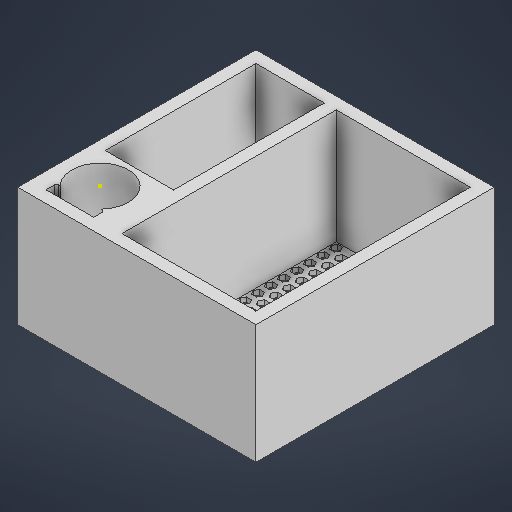
# Autodesk Inventor part: mount
Saved by Autodesk Inventor 2026.1 (Build 301233020, 233B)
## iProperties
Created: 2025-12-18
Part Number: mount
Material: Generic
Document SubType Name: Modeling
Designer: Fish
Density: 1 g/cm^3
Appearance: Default
Author: Fish
Autodesk Inventor part; units mm, degrees
(part 1 of 4)
ref_plane "YZ Plane" through (0, 0, 0) normal (1, 0, 0) x (0, 1, 0)
ref_plane "XZ Plane" through (0, 0, 0) normal (0, 1, 0) x (-1, 0, 0)
ref_plane "XY Plane" through (0, 0, 0) normal (0, 0, 1) x (1, 0, 0)
sketch "Sketch1" plane through (0, 0, 0) normal (0, 1, 0) x (-1, 0, 0)
  circle A0 centre (0, 0) radius 11.5
  circle A1 centre (0, 0) radius 11.85
  line L0 (10, 12.5) -> (-10, 12.5)
  line L1 (-10, 12.5) -> (-10, 8.2614)
  line L2 (-10, 8.2614) -> (10, 8.2614)
  line L3 (10, 8.2614) -> (10, 12.5)
  line L4 (10, 12.5) -> (-10, 8.2614) construction
  line L5 (-10, 12.5) -> (10, 8.2614) construction
  line L6 (0, 10.3807) -> (0, -11.5) construction
  line L7 (10, 12.5) -> (-10, 12.5)
  line L8 (-10, 12.5) -> (-10, 12.7)
  line L9 (-10, 12.7) -> (10, 12.7)
  line L10 (10, 12.7) -> (10, 12.5)
  line L11 (-16.85, 17.7) -> (16.85, 17.7)
  line L12 (16.85, 17.7) -> (16.85, -14)
  line L13 (16.85, -14) -> (-16.85, -14)
  line L14 (-16.85, -14) -> (-16.85, 17.7)
  point P0 (8, 8.2614)
  point P1 (-8, 8.2614)
  point P2 (0, -14)
  point P3 (8.4954, 8.2614)
  point P4 (-8.4954, 8.2614)
  dimension "d0" = 23
  dimension "d1" = 0.35
  dimension "d2" = 24
  dimension "d3" = 16
  dimension "d4" = 20
  dimension "d5" = 0.2
  dimension "d6" = 5
  dimension "d7" = 2.5
  dimension "d8" = 5
  dimension "d9" = 16.85
  dimension "d10" = 16.85
  constraints: 30 end point, 6 parallel, 3 horizontal, 3 midpoint, 3 perpendicular, 3 point on circle, 3 point on line, 2 centre point, 2 coincident, 1 vertical
  measures "d0" diameter of A0
  measures "d1" radial gap between concentric circles of A1 A0
  measures "d2" distance from line of L0 L6.end
  measures "d3" distance of point (-8, 8.261) A0.end
  measures "d4" distance of L0.start L0.end
  measures "d5" distance between parallel lines of L9 L0
  measures "d6" distance between parallel lines of L11 L9
  measures "d7" distance of point (0, -14) L6.end
  measures "d8" distance edge to line of A1 L14
  measures "d9" distance between parallel lines of L14 L6
  measures "d10" distance between parallel lines of L12 L6
extrude "Extrusion1" add sketch "Sketch1" along normal blind 50
fillet "Fillet1" radius 0.25 2 edges at (8.4954, 25, 8.2614) (-8.4954, 25, 8.2614)
chamfer "Chamfer1" distance 0.75 angle 45 2 edges at (-10, 25, 8.2614) (10, 25, 8.2614)
sketch "Sketch2" plane through (16.85, 0, -14) normal (0, 0, -1) x (-1, 0, 0)
  line L0 (5, 50) -> (28.7, 50) projected
  line L1 (5, 50) -> (28.7, 50)
  line L2 (28.7, 50) -> (28.7, 0)
  line L3 (28.7, 0) -> (5, 0)
  line L4 (5, 0) -> (5, 50)
  line L5 (0, 0) -> (33.7, 0) projected
  circle A0 centre (8.8, 2.3324) radius 3.5
  circle A1 centre (8.8, 2.3324) radius 3.8
  line L6 (5.8, 0) -> (11.8, 0) construction
  line L7 (5.3, 0) -> (5.3, 50)
  point P0 (16.85, 0)
  point P1 (25.7306, 50)
  point P2 (7.9694, 50)
  point P3 (2.5, 2.3324)
  point P4 (6.1904, 0)
  point P5 (11.8, 0)
  point P6 (5, 2.3324)
  point P7 (2.5, 0.8525)
  point P8 (11.4096, 0)
  dimension "d17" = 7
  dimension "d18" = 0.3
  dimension "d20" = 6
  dimension "d25" = 0.3
  constraints: 12 end point, 4 point on line, 2 centre point, 2 horizontal, 2 parallel, 2 perpendicular, 2 point on circle, 1 coincident, 1 tangent
  measures "d17" diameter of A0
  measures "d18" radial gap between concentric circles of A1 A0
  measures "d20" distance of L6.end L6.start
  measures "d25" distance between parallel lines of L4 L7
extrude "Extrusion2" cut sketch "Sketch2" against normal up to surface contours A1 L7 | A1 L3 A0 L7 | L7 A0 L3 A1 | A0 L3 | L3 A0 A1 | L3 A0
fillet "Fillet2" radius 0.25 2 edges at (5.05, 0, -12.36) (11.05, 0, -9.1401)
sketch "Sketch4" plane through (16.85, 50, -14) normal (0, 0, -1) x (-1, 0, 0)
  arc A0 (5.3264, -50) -> (5.5408, -49.6215) centre (5.3264, -49.75) ccw projected
  arc A1 (12.0592, -49.6215) -> (5.5408, -49.6215) centre (8.8, -47.6676) ccw projected
  arc A2 (12.0592, -49.6215) -> (12.2736, -50) centre (12.2736, -49.75) ccw projected
  line L0 (12.2736, -50) -> (33.7, -50) projected
  line L1 (33.7, -50) -> (33.7, 0) projected
  line L2 (0, 0) -> (33.7, 0) projected
  line L3 (0, -50) -> (0, 0) projected
  line L4 (0, -50) -> (5.3264, -50) projected
  line L5 (5.5764, -49.0955) -> (12.0236, -49.0955)
  line L6 (12.0236, -49.0955) -> (12.0236, -49.986)
  line L7 (12.0236, -49.986) -> (5.5764, -49.986)
  line L8 (5.5764, -49.986) -> (5.5764, -49.0955)
  arc A3 (12.0592, -49.6215) -> (12.2736, -50) centre (12.2736, -49.75) ccw projected
  point P0 (16.85, -50)
  dimension "d26" = 6.4473
  constraints: 8 end point, 2 parallel, 2 tangent, 1 horizontal, 1 perpendicular
  measures "d26" distance of L5.start L5.end
sketch "Sketch5" plane through (0, 50, 0) normal (0, 1, 0) x (1, 0, 0)
  point P0 (0, 0)
sketch "Sketch6" plane through (0, 50, 0) normal (0, 1, 0) x (1, 0, 0)
  line L0 (-16.85, -17.7) -> (16.85, -17.7) projected
  line L1 (-16.85, -17.7) -> (83.15, -17.7)
  line L2 (83.15, -17.7) -> (83.15, 82.3)
  line L3 (83.15, 82.3) -> (-16.85, 82.3)
  line L4 (-16.85, 82.3) -> (-16.85, -17.7)
  line L5 (16.85, -17.7) -> (16.85, 14) projected
  line L6 (16.85, -17.7) -> (21.85, -17.7)
  line L7 (21.85, -17.7) -> (21.85, 82.3)
  line L8 (21.85, 82.3) -> (16.85, 82.3)
  line L9 (16.85, 82.3) -> (16.85, -17.7)
  line L10 (21.85, -17.7) -> (83.15, -17.7)
  line L11 (83.15, -17.7) -> (83.15, -12.7)
  line L12 (83.15, -12.7) -> (21.85, -12.7)
  line L13 (21.85, -12.7) -> (21.85, -17.7)
  line L14 (21.85, 82.3) -> (83.15, 82.3)
  line L15 (83.15, 82.3) -> (83.15, 77.3)
  line L16 (83.15, 77.3) -> (21.85, 77.3)
  line L17 (21.85, 77.3) -> (21.85, 82.3)
  line L18 (83.15, -12.7) -> (78.15, -12.7)
  line L19 (78.15, -12.7) -> (78.15, 77.3)
  line L20 (78.15, 77.3) -> (83.15, 77.3)
  line L21 (83.15, 77.3) -> (83.15, -12.7)
  line L22 (16.85, 14) -> (-16.85, 14) projected
  line L23 (-16.85, 14) -> (-11.85, 14)
  line L24 (-11.85, 14) -> (-11.85, 82.3)
  line L25 (-11.85, 82.3) -> (-16.85, 82.3)
  line L26 (-16.85, 82.3) -> (-16.85, 14)
  line L27 (-11.85, 82.3) -> (21.85, 82.3)
  line L28 (21.85, 82.3) -> (21.85, 77.3)
  line L29 (21.85, 77.3) -> (-11.85, 77.3)
  line L30 (-11.85, 77.3) -> (-11.85, 82.3)
  point P0 (0, 0)
  point P1 (-11.85, 77.3)
  point P2 (16.85, 77.3)
  point P3 (16.85, -17.7)
  dimension "d29" = 5
  dimension "d30" = 5
  dimension "d31" = 100
  dimension "d32" = 100
  dimension "d33" = 5
  dimension "d34" = 5
  dimension "d35" = 5
  constraints: 56 end point, 14 parallel, 7 horizontal, 7 perpendicular, 5 point on line
  measures "d29" distance between parallel lines of L7 L9
  measures "d30" distance between parallel lines of L1 L12
  measures "d31" distance of L3.end L0.start
  measures "d32" distance of L2.end L3.end
  measures "d33" distance between parallel lines of L3 L16
  measures "d34" distance between parallel lines of L21 L19
  measures "d35" distance between parallel lines of L4 L24
extrude "Extrusion3" add sketch "Sketch6" against normal up to surface (50 mm away) contours L5 L9 L29 L7 L1 | L4 L3 L24 L22 | L7 L12 L2 L1 | L29 L24 L3 L9 | L9 L3 L7 L29 | L12 L19 L16 L2 | L7 L3 L2 L16
sketch "Sketch7" plane through (0, 0, 0) normal (0, -1, 0) x (1, 0, 0)
  line L0 (21.85, -77.3) -> (21.85, 12.7) projected
  line L1 (21.85, 12.7) -> (78.15, 12.7) projected
  line L2 (78.15, 12.7) -> (78.15, -77.3) projected
  line L3 (78.15, -77.3) -> (21.85, -77.3) projected
  line L4 (20.35, 16.9321) -> (21.35, 15.2)
  line L5 (21.35, 15.2) -> (20.35, 13.4679)
  line L6 (20.35, 13.4679) -> (18.35, 13.4679)
  line L7 (18.35, 13.4679) -> (17.35, 15.2)
  line L8 (17.35, 15.2) -> (18.35, 16.9321)
  line L9 (18.35, 16.9321) -> (20.35, 16.9321)
  line L10 (-16.85, 17.7) -> (83.15, 17.7) projected
  line L11 (25.0821, 19.6641) -> (26.0821, 17.9321)
  line L12 (26.0821, 17.9321) -> (25.0821, 16.2)
  line L13 (25.0821, 16.2) -> (23.0821, 16.2)
  line L14 (23.0821, 16.2) -> (22.0821, 17.9321)
  line L15 (22.0821, 17.9321) -> (23.0821, 19.6641)
  line L16 (23.0821, 19.6641) -> (25.0821, 19.6641)
  line L17 (29.8141, 16.9321) -> (30.8141, 15.2)
  line L18 (30.8141, 15.2) -> (29.8141, 13.4679)
  line L19 (29.8141, 13.4679) -> (27.8141, 13.4679)
  line L20 (27.8141, 13.4679) -> (26.8141, 15.2)
  line L21 (26.8141, 15.2) -> (27.8141, 16.9321)
  line L22 (27.8141, 16.9321) -> (29.8141, 16.9321)
  line L23 (20.35, 16.9321) -> (22.0821, 17.9321) construction
  line L24 (25.0821, 16.2) -> (26.8141, 15.2) construction
  line L25 (25.0821, 14.2) -> (26.0821, 12.4679)
  line L26 (26.0821, 12.4679) -> (25.0821, 10.7359)
  line L27 (25.0821, 10.7359) -> (23.0821, 10.7359)
  line L28 (23.0821, 10.7359) -> (22.0821, 12.4679)
  line L29 (22.0821, 12.4679) -> (23.0821, 14.2)
  line L30 (23.0821, 14.2) -> (25.0821, 14.2)
  line L31 (20.35, 11.4679) -> (21.35, 9.7359)
  line L32 (21.35, 9.7359) -> (20.35, 8.0038)
  line L33 (20.35, 8.0038) -> (18.35, 8.0038)
  line L34 (18.35, 8.0038) -> (17.35, 9.7359)
  line L35 (17.35, 9.7359) -> (18.35, 11.4679)
  line L36 (18.35, 11.4679) -> (20.35, 11.4679)
  line L37 (18.35, 13.4679) -> (18.35, 11.4679) construction
  line L38 (27.8141, 13.4679) -> (26.8141, 15.2)
  line L39 (30.8141, 15.2) -> (29.8141, 13.4679)
  line L40 (27.8141, 16.9321) -> (29.8141, 16.9321)
  line L41 (29.8141, 16.9321) -> (30.8141, 15.2)
  line L42 (29.8141, 13.4679) -> (27.8141, 13.4679)
  line L43 (26.8141, 15.2) -> (27.8141, 16.9321)
  line L44 (32.5462, 16.2) -> (31.5462, 17.9321)
  line L45 (34.5462, 16.2) -> (32.5462, 16.2)
  line L46 (35.5462, 17.9321) -> (34.5462, 16.2)
  line L47 (31.5462, 17.9321) -> (32.5462, 19.6641)
  line L48 (32.5462, 19.6641) -> (34.5462, 19.6641)
  line L49 (34.5462, 19.6641) -> (35.5462, 17.9321)
  line L50 (37.2782, 13.4679) -> (36.2782, 15.2)
  line L51 (40.2782, 15.2) -> (39.2782, 13.4679)
  line L52 (37.2782, 16.9321) -> (39.2782, 16.9321)
  line L53 (39.2782, 16.9321) -> (40.2782, 15.2)
  line L54 (39.2782, 13.4679) -> (37.2782, 13.4679)
  line L55 (36.2782, 15.2) -> (37.2782, 16.9321)
  line L56 (42.0103, 16.2) -> (41.0103, 17.9321)
  line L57 (44.0103, 16.2) -> (42.0103, 16.2)
  line L58 (45.0103, 17.9321) -> (44.0103, 16.2)
  line L59 (41.0103, 17.9321) -> (42.0103, 19.6641)
  line L60 (42.0103, 19.6641) -> (44.0103, 19.6641)
  line L61 (44.0103, 19.6641) -> (45.0103, 17.9321)
  line L62 (46.7423, 13.4679) -> (45.7423, 15.2)
  line L63 (49.7423, 15.2) -> (48.7423, 13.4679)
  line L64 (46.7423, 16.9321) -> (48.7423, 16.9321)
  line L65 (48.7423, 16.9321) -> (49.7423, 15.2)
  line L66 (48.7423, 13.4679) -> (46.7423, 13.4679)
  line L67 (45.7423, 15.2) -> (46.7423, 16.9321)
  line L68 (51.4744, 16.2) -> (50.4744, 17.9321)
  line L69 (53.4744, 16.2) -> (51.4744, 16.2)
  line L70 (54.4744, 17.9321) -> (53.4744, 16.2)
  line L71 (50.4744, 17.9321) -> (51.4744, 19.6641)
  line L72 (51.4744, 19.6641) -> (53.4744, 19.6641)
  line L73 (53.4744, 19.6641) -> (54.4744, 17.9321)
  line L74 (56.2064, 13.4679) -> (55.2064, 15.2)
  line L75 (59.2064, 15.2) -> (58.2064, 13.4679)
  line L76 (56.2064, 16.9321) -> (58.2064, 16.9321)
  line L77 (58.2064, 16.9321) -> (59.2064, 15.2)
  line L78 (58.2064, 13.4679) -> (56.2064, 13.4679)
  line L79 (55.2064, 15.2) -> (56.2064, 16.9321)
  line L80 (60.9385, 16.2) -> (59.9385, 17.9321)
  line L81 (62.9385, 16.2) -> (60.9385, 16.2)
  line L82 (63.9385, 17.9321) -> (62.9385, 16.2)
  line L83 (59.9385, 17.9321) -> (60.9385, 19.6641)
  line L84 (60.9385, 19.6641) -> (62.9385, 19.6641)
  line L85 (62.9385, 19.6641) -> (63.9385, 17.9321)
  line L86 (65.6705, 13.4679) -> (64.6705, 15.2)
  line L87 (68.6705, 15.2) -> (67.6705, 13.4679)
  line L88 (65.6705, 16.9321) -> (67.6705, 16.9321)
  line L89 (67.6705, 16.9321) -> (68.6705, 15.2)
  line L90 (67.6705, 13.4679) -> (65.6705, 13.4679)
  line L91 (64.6705, 15.2) -> (65.6705, 16.9321)
  line L92 (70.4026, 16.2) -> (69.4026, 17.9321)
  line L93 (72.4026, 16.2) -> (70.4026, 16.2)
  line L94 (73.4026, 17.9321) -> (72.4026, 16.2)
  line L95 (69.4026, 17.9321) -> (70.4026, 19.6641)
  line L96 (70.4026, 19.6641) -> (72.4026, 19.6641)
  line L97 (72.4026, 19.6641) -> (73.4026, 17.9321)
  line L98 (75.1346, 13.4679) -> (74.1346, 15.2)
  line L99 (78.1346, 15.2) -> (77.1346, 13.4679)
  line L100 (75.1346, 16.9321) -> (77.1346, 16.9321)
  line L101 (77.1346, 16.9321) -> (78.1346, 15.2)
  line L102 (77.1346, 13.4679) -> (75.1346, 13.4679)
  line L103 (74.1346, 15.2) -> (75.1346, 16.9321)
  line L104 (79.8667, 16.2) -> (78.8667, 17.9321)
  line L105 (81.8667, 16.2) -> (79.8667, 16.2)
  line L106 (82.8667, 17.9321) -> (81.8667, 16.2)
  line L107 (78.8667, 17.9321) -> (79.8667, 19.6641)
  line L108 (79.8667, 19.6641) -> (81.8667, 19.6641)
  line L109 (81.8667, 19.6641) -> (82.8667, 17.9321)
  line L110 (18.35, 8.0038) -> (17.35, 9.7359)
  line L111 (21.35, 9.7359) -> (20.35, 8.0038)
  line L112 (18.35, 11.4679) -> (20.35, 11.4679)
  line L113 (20.35, 11.4679) -> (21.35, 9.7359)
  line L114 (20.35, 8.0038) -> (18.35, 8.0038)
  line L115 (17.35, 9.7359) -> (18.35, 11.4679)
  line L116 (23.0821, 10.7359) -> (22.0821, 12.4679)
  line L117 (25.0821, 10.7359) -> (23.0821, 10.7359)
  line L118 (26.0821, 12.4679) -> (25.0821, 10.7359)
  line L119 (22.0821, 12.4679) -> (23.0821, 14.2)
  line L120 (23.0821, 14.2) -> (25.0821, 14.2)
  line L121 (25.0821, 14.2) -> (26.0821, 12.4679)
  line L122 (27.8141, 8.0038) -> (26.8141, 9.7359)
  line L123 (30.8141, 9.7359) -> (29.8141, 8.0038)
  line L124 (27.8141, 11.4679) -> (29.8141, 11.4679)
  line L125 (29.8141, 11.4679) -> (30.8141, 9.7359)
  line L126 (29.8141, 8.0038) -> (27.8141, 8.0038)
  line L127 (26.8141, 9.7359) -> (27.8141, 11.4679)
  line L128 (32.5462, 10.7359) -> (31.5462, 12.4679)
  line L129 (34.5462, 10.7359) -> (32.5462, 10.7359)
  line L130 (35.5462, 12.4679) -> (34.5462, 10.7359)
  line L131 (31.5462, 12.4679) -> (32.5462, 14.2)
  line L132 (32.5462, 14.2) -> (34.5462, 14.2)
  line L133 (34.5462, 14.2) -> (35.5462, 12.4679)
  line L134 (37.2782, 8.0038) -> (36.2782, 9.7359)
  line L135 (40.2782, 9.7359) -> (39.2782, 8.0038)
  line L136 (37.2782, 11.4679) -> (39.2782, 11.4679)
  line L137 (39.2782, 11.4679) -> (40.2782, 9.7359)
  line L138 (39.2782, 8.0038) -> (37.2782, 8.0038)
  line L139 (36.2782, 9.7359) -> (37.2782, 11.4679)
  line L140 (42.0103, 10.7359) -> (41.0103, 12.4679)
  line L141 (44.0103, 10.7359) -> (42.0103, 10.7359)
  line L142 (45.0103, 12.4679) -> (44.0103, 10.7359)
  line L143 (41.0103, 12.4679) -> (42.0103, 14.2)
  line L144 (42.0103, 14.2) -> (44.0103, 14.2)
  line L145 (44.0103, 14.2) -> (45.0103, 12.4679)
  line L146 (46.7423, 8.0038) -> (45.7423, 9.7359)
  line L147 (49.7423, 9.7359) -> (48.7423, 8.0038)
  line L148 (46.7423, 11.4679) -> (48.7423, 11.4679)
  line L149 (48.7423, 11.4679) -> (49.7423, 9.7359)
  line L150 (48.7423, 8.0038) -> (46.7423, 8.0038)
  line L151 (45.7423, 9.7359) -> (46.7423, 11.4679)
  line L152 (51.4744, 10.7359) -> (50.4744, 12.4679)
  line L153 (53.4744, 10.7359) -> (51.4744, 10.7359)
  line L154 (54.4744, 12.4679) -> (53.4744, 10.7359)
  line L155 (50.4744, 12.4679) -> (51.4744, 14.2)
  line L156 (51.4744, 14.2) -> (53.4744, 14.2)
  line L157 (53.4744, 14.2) -> (54.4744, 12.4679)
  line L158 (56.2064, 8.0038) -> (55.2064, 9.7359)
  line L159 (59.2064, 9.7359) -> (58.2064, 8.0038)
  line L160 (56.2064, 11.4679) -> (58.2064, 11.4679)
  line L161 (58.2064, 11.4679) -> (59.2064, 9.7359)
  line L162 (58.2064, 8.0038) -> (56.2064, 8.0038)
  line L163 (55.2064, 9.7359) -> (56.2064, 11.4679)
  line L164 (60.9385, 10.7359) -> (59.9385, 12.4679)
  line L165 (62.9385, 10.7359) -> (60.9385, 10.7359)
  line L166 (63.9385, 12.4679) -> (62.9385, 10.7359)
  line L167 (59.9385, 12.4679) -> (60.9385, 14.2)
  line L168 (60.9385, 14.2) -> (62.9385, 14.2)
  line L169 (62.9385, 14.2) -> (63.9385, 12.4679)
  line L170 (65.6705, 8.0038) -> (64.6705, 9.7359)
  line L171 (68.6705, 9.7359) -> (67.6705, 8.0038)
  line L172 (65.6705, 11.4679) -> (67.6705, 11.4679)
  line L173 (67.6705, 11.4679) -> (68.6705, 9.7359)
  line L174 (67.6705, 8.0038) -> (65.6705, 8.0038)
  line L175 (64.6705, 9.7359) -> (65.6705, 11.4679)
  line L176 (70.4026, 10.7359) -> (69.4026, 12.4679)
  line L177 (72.4026, 10.7359) -> (70.4026, 10.7359)
  line L178 (73.4026, 12.4679) -> (72.4026, 10.7359)
  line L179 (69.4026, 12.4679) -> (70.4026, 14.2)
  line L180 (70.4026, 14.2) -> (72.4026, 14.2)
  line L181 (72.4026, 14.2) -> (73.4026, 12.4679)
  line L182 (75.1346, 8.0038) -> (74.1346, 9.7359)
  line L183 (78.1346, 9.7359) -> (77.1346, 8.0038)
  line L184 (75.1346, 11.4679) -> (77.1346, 11.4679)
  line L185 (77.1346, 11.4679) -> (78.1346, 9.7359)
  line L186 (77.1346, 8.0038) -> (75.1346, 8.0038)
  line L187 (74.1346, 9.7359) -> (75.1346, 11.4679)
  line L188 (79.8667, 10.7359) -> (78.8667, 12.4679)
  line L189 (81.8667, 10.7359) -> (79.8667, 10.7359)
  line L190 (82.8667, 12.4679) -> (81.8667, 10.7359)
  line L191 (78.8667, 12.4679) -> (79.8667, 14.2)
  line L192 (79.8667, 14.2) -> (81.8667, 14.2)
  line L193 (81.8667, 14.2) -> (82.8667, 12.4679)
  line L194 (18.35, 2.5397) -> (17.35, 4.2718)
  line L195 (21.35, 4.2718) -> (20.35, 2.5397)
  line L196 (18.35, 6.0038) -> (20.35, 6.0038)
  line L197 (20.35, 6.0038) -> (21.35, 4.2718)
  line L198 (20.35, 2.5397) -> (18.35, 2.5397)
  line L199 (17.35, 4.2718) -> (18.35, 6.0038)
  line L200 (23.0821, 5.2718) -> (22.0821, 7.0038)
  line L201 (25.0821, 5.2718) -> (23.0821, 5.2718)
  line L202 (26.0821, 7.0038) -> (25.0821, 5.2718)
  line L203 (22.0821, 7.0038) -> (23.0821, 8.7359)
  line L204 (23.0821, 8.7359) -> (25.0821, 8.7359)
  line L205 (25.0821, 8.7359) -> (26.0821, 7.0038)
  line L206 (27.8141, 2.5397) -> (26.8141, 4.2718)
  line L207 (30.8141, 4.2718) -> (29.8141, 2.5397)
  line L208 (27.8141, 6.0038) -> (29.8141, 6.0038)
  line L209 (29.8141, 6.0038) -> (30.8141, 4.2718)
  line L210 (29.8141, 2.5397) -> (27.8141, 2.5397)
  line L211 (26.8141, 4.2718) -> (27.8141, 6.0038)
  line L212 (32.5462, 5.2718) -> (31.5462, 7.0038)
  line L213 (34.5462, 5.2718) -> (32.5462, 5.2718)
  line L214 (35.5462, 7.0038) -> (34.5462, 5.2718)
  line L215 (31.5462, 7.0038) -> (32.5462, 8.7359)
  line L216 (32.5462, 8.7359) -> (34.5462, 8.7359)
  line L217 (34.5462, 8.7359) -> (35.5462, 7.0038)
  line L218 (37.2782, 2.5397) -> (36.2782, 4.2718)
  line L219 (40.2782, 4.2718) -> (39.2782, 2.5397)
  line L220 (37.2782, 6.0038) -> (39.2782, 6.0038)
  line L221 (39.2782, 6.0038) -> (40.2782, 4.2718)
  line L222 (39.2782, 2.5397) -> (37.2782, 2.5397)
  line L223 (36.2782, 4.2718) -> (37.2782, 6.0038)
  line L224 (42.0103, 5.2718) -> (41.0103, 7.0038)
  line L225 (44.0103, 5.2718) -> (42.0103, 5.2718)
  line L226 (45.0103, 7.0038) -> (44.0103, 5.2718)
  line L227 (41.0103, 7.0038) -> (42.0103, 8.7359)
  line L228 (42.0103, 8.7359) -> (44.0103, 8.7359)
  line L229 (44.0103, 8.7359) -> (45.0103, 7.0038)
  line L230 (46.7423, 2.5397) -> (45.7423, 4.2718)
  line L231 (49.7423, 4.2718) -> (48.7423, 2.5397)
  line L232 (46.7423, 6.0038) -> (48.7423, 6.0038)
  line L233 (48.7423, 6.0038) -> (49.7423, 4.2718)
  line L234 (48.7423, 2.5397) -> (46.7423, 2.5397)
  line L235 (45.7423, 4.2718) -> (46.7423, 6.0038)
  line L236 (51.4744, 5.2718) -> (50.4744, 7.0038)
  line L237 (53.4744, 5.2718) -> (51.4744, 5.2718)
  line L238 (54.4744, 7.0038) -> (53.4744, 5.2718)
  line L239 (50.4744, 7.0038) -> (51.4744, 8.7359)
  line L240 (51.4744, 8.7359) -> (53.4744, 8.7359)
  line L241 (53.4744, 8.7359) -> (54.4744, 7.0038)
  line L242 (56.2064, 2.5397) -> (55.2064, 4.2718)
  line L243 (59.2064, 4.2718) -> (58.2064, 2.5397)
  line L244 (56.2064, 6.0038) -> (58.2064, 6.0038)
  line L245 (58.2064, 6.0038) -> (59.2064, 4.2718)
  line L246 (58.2064, 2.5397) -> (56.2064, 2.5397)
  line L247 (55.2064, 4.2718) -> (56.2064, 6.0038)
  line L248 (60.9385, 5.2718) -> (59.9385, 7.0038)
  line L249 (62.9385, 5.2718) -> (60.9385, 5.2718)
  line L250 (63.9385, 7.0038) -> (62.9385, 5.2718)
  line L251 (59.9385, 7.0038) -> (60.9385, 8.7359)
  line L252 (60.9385, 8.7359) -> (62.9385, 8.7359)
  line L253 (62.9385, 8.7359) -> (63.9385, 7.0038)
  line L254 (65.6705, 2.5397) -> (64.6705, 4.2718)
  line L255 (68.6705, 4.2718) -> (67.6705, 2.5397)
  line L256 (65.6705, 6.0038) -> (67.6705, 6.0038)
  line L257 (67.6705, 6.0038) -> (68.6705, 4.2718)
  line L258 (67.6705, 2.5397) -> (65.6705, 2.5397)
  line L259 (64.6705, 4.2718) -> (65.6705, 6.0038)
  line L260 (70.4026, 5.2718) -> (69.4026, 7.0038)
  line L261 (72.4026, 5.2718) -> (70.4026, 5.2718)
  line L262 (73.4026, 7.0038) -> (72.4026, 5.2718)
  line L263 (69.4026, 7.0038) -> (70.4026, 8.7359)
  line L264 (70.4026, 8.7359) -> (72.4026, 8.7359)
  line L265 (72.4026, 8.7359) -> (73.4026, 7.0038)
  line L266 (75.1346, 2.5397) -> (74.1346, 4.2718)
  line L267 (78.1346, 4.2718) -> (77.1346, 2.5397)
  line L268 (75.1346, 6.0038) -> (77.1346, 6.0038)
  line L269 (77.1346, 6.0038) -> (78.1346, 4.2718)
  line L270 (77.1346, 2.5397) -> (75.1346, 2.5397)
  line L271 (74.1346, 4.2718) -> (75.1346, 6.0038)
  line L272 (79.8667, 5.2718) -> (78.8667, 7.0038)
  line L273 (81.8667, 5.2718) -> (79.8667, 5.2718)
  line L274 (82.8667, 7.0038) -> (81.8667, 5.2718)
  line L275 (78.8667, 7.0038) -> (79.8667, 8.7359)
  line L276 (79.8667, 8.7359) -> (81.8667, 8.7359)
  line L277 (81.8667, 8.7359) -> (82.8667, 7.0038)
  line L278 (18.35, -2.9244) -> (17.35, -1.1923)
  line L279 (21.35, -1.1923) -> (20.35, -2.9244)
  line L280 (18.35, 0.5397) -> (20.35, 0.5397)
  line L281 (20.35, 0.5397) -> (21.35, -1.1923)
  line L282 (20.35, -2.9244) -> (18.35, -2.9244)
  line L283 (17.35, -1.1923) -> (18.35, 0.5397)
  line L284 (23.0821, -0.1923) -> (22.0821, 1.5397)
  line L285 (25.0821, -0.1923) -> (23.0821, -0.1923)
  line L286 (26.0821, 1.5397) -> (25.0821, -0.1923)
  line L287 (22.0821, 1.5397) -> (23.0821, 3.2718)
  line L288 (23.0821, 3.2718) -> (25.0821, 3.2718)
  line L289 (25.0821, 3.2718) -> (26.0821, 1.5397)
  line L290 (27.8141, -2.9244) -> (26.8141, -1.1923)
  line L291 (30.8141, -1.1923) -> (29.8141, -2.9244)
  line L292 (27.8141, 0.5397) -> (29.8141, 0.5397)
  line L293 (29.8141, 0.5397) -> (30.8141, -1.1923)
  line L294 (29.8141, -2.9244) -> (27.8141, -2.9244)
  line L295 (26.8141, -1.1923) -> (27.8141, 0.5397)
  line L296 (32.5462, -0.1923) -> (31.5462, 1.5397)
  line L297 (34.5462, -0.1923) -> (32.5462, -0.1923)
  line L298 (35.5462, 1.5397) -> (34.5462, -0.1923)
  line L299 (31.5462, 1.5397) -> (32.5462, 3.2718)
  line L300 (32.5462, 3.2718) -> (34.5462, 3.2718)
  line L301 (34.5462, 3.2718) -> (35.5462, 1.5397)
  line L302 (37.2782, -2.9244) -> (36.2782, -1.1923)
  line L303 (40.2782, -1.1923) -> (39.2782, -2.9244)
  line L304 (37.2782, 0.5397) -> (39.2782, 0.5397)
  line L305 (39.2782, 0.5397) -> (40.2782, -1.1923)
  line L306 (39.2782, -2.9244) -> (37.2782, -2.9244)
  line L307 (36.2782, -1.1923) -> (37.2782, 0.5397)
  line L308 (42.0103, -0.1923) -> (41.0103, 1.5397)
  line L309 (44.0103, -0.1923) -> (42.0103, -0.1923)
  line L310 (45.0103, 1.5397) -> (44.0103, -0.1923)
  line L311 (41.0103, 1.5397) -> (42.0103, 3.2718)
  line L312 (42.0103, 3.2718) -> (44.0103, 3.2718)
  line L313 (44.0103, 3.2718) -> (45.0103, 1.5397)
  line L314 (46.7423, -2.9244) -> (45.7423, -1.1923)
  line L315 (49.7423, -1.1923) -> (48.7423, -2.9244)
  line L316 (46.7423, 0.5397) -> (48.7423, 0.5397)
  line L317 (48.7423, 0.5397) -> (49.7423, -1.1923)
  line L318 (48.7423, -2.9244) -> (46.7423, -2.9244)
  line L319 (45.7423, -1.1923) -> (46.7423, 0.5397)
  line L320 (51.4744, -0.1923) -> (50.4744, 1.5397)
  line L321 (53.4744, -0.1923) -> (51.4744, -0.1923)
  line L322 (54.4744, 1.5397) -> (53.4744, -0.1923)
  line L323 (50.4744, 1.5397) -> (51.4744, 3.2718)
  line L324 (51.4744, 3.2718) -> (53.4744, 3.2718)
  line L325 (53.4744, 3.2718) -> (54.4744, 1.5397)
  line L326 (56.2064, -2.9244) -> (55.2064, -1.1923)
  line L327 (59.2064, -1.1923) -> (58.2064, -2.9244)
  line L328 (56.2064, 0.5397) -> (58.2064, 0.5397)
  line L329 (58.2064, 0.5397) -> (59.2064, -1.1923)
  line L330 (58.2064, -2.9244) -> (56.2064, -2.9244)
  line L331 (55.2064, -1.1923) -> (56.2064, 0.5397)
  line L332 (60.9385, -0.1923) -> (59.9385, 1.5397)
  line L333 (62.9385, -0.1923) -> (60.9385, -0.1923)
  line L334 (63.9385, 1.5397) -> (62.9385, -0.1923)
  line L335 (59.9385, 1.5397) -> (60.9385, 3.2718)
  line L336 (60.9385, 3.2718) -> (62.9385, 3.2718)
  line L337 (62.9385, 3.2718) -> (63.9385, 1.5397)
  line L338 (65.6705, -2.9244) -> (64.6705, -1.1923)
  line L339 (68.6705, -1.1923) -> (67.6705, -2.9244)
  line L340 (65.6705, 0.5397) -> (67.6705, 0.5397)
  line L341 (67.6705, 0.5397) -> (68.6705, -1.1923)
  line L342 (67.6705, -2.9244) -> (65.6705, -2.9244)
  line L343 (64.6705, -1.1923) -> (65.6705, 0.5397)
  line L344 (70.4026, -0.1923) -> (69.4026, 1.5397)
  line L345 (72.4026, -0.1923) -> (70.4026, -0.1923)
  line L346 (73.4026, 1.5397) -> (72.4026, -0.1923)
  line L347 (69.4026, 1.5397) -> (70.4026, 3.2718)
  line L348 (70.4026, 3.2718) -> (72.4026, 3.2718)
  line L349 (72.4026, 3.2718) -> (73.4026, 1.5397)
  line L350 (75.1346, -2.9244) -> (74.1346, -1.1923)
  line L351 (78.1346, -1.1923) -> (77.1346, -2.9244)
  line L352 (75.1346, 0.5397) -> (77.1346, 0.5397)
  line L353 (77.1346, 0.5397) -> (78.1346, -1.1923)
  line L354 (77.1346, -2.9244) -> (75.1346, -2.9244)
  line L355 (74.1346, -1.1923) -> (75.1346, 0.5397)
  line L356 (79.8667, -0.1923) -> (78.8667, 1.5397)
  line L357 (81.8667, -0.1923) -> (79.8667, -0.1923)
  line L358 (82.8667, 1.5397) -> (81.8667, -0.1923)
  line L359 (78.8667, 1.5397) -> (79.8667, 3.2718)
  line L360 (79.8667, 3.2718) -> (81.8667, 3.2718)
  line L361 (81.8667, 3.2718) -> (82.8667, 1.5397)
  line L362 (18.35, -8.3885) -> (17.35, -6.6564)
  line L363 (21.35, -6.6564) -> (20.35, -8.3885)
  line L364 (18.35, -4.9244) -> (20.35, -4.9244)
  line L365 (20.35, -4.9244) -> (21.35, -6.6564)
  line L366 (20.35, -8.3885) -> (18.35, -8.3885)
  line L367 (17.35, -6.6564) -> (18.35, -4.9244)
  line L368 (23.0821, -5.6564) -> (22.0821, -3.9244)
  line L369 (25.0821, -5.6564) -> (23.0821, -5.6564)
  line L370 (26.0821, -3.9244) -> (25.0821, -5.6564)
  line L371 (22.0821, -3.9244) -> (23.0821, -2.1923)
  line L372 (23.0821, -2.1923) -> (25.0821, -2.1923)
  line L373 (25.0821, -2.1923) -> (26.0821, -3.9244)
  line L374 (27.8141, -8.3885) -> (26.8141, -6.6564)
  line L375 (30.8141, -6.6564) -> (29.8141, -8.3885)
  line L376 (27.8141, -4.9244) -> (29.8141, -4.9244)
  line L377 (29.8141, -4.9244) -> (30.8141, -6.6564)
  line L378 (29.8141, -8.3885) -> (27.8141, -8.3885)
  line L379 (26.8141, -6.6564) -> (27.8141, -4.9244)
  line L380 (32.5462, -5.6564) -> (31.5462, -3.9244)
  line L381 (34.5462, -5.6564) -> (32.5462, -5.6564)
  line L382 (35.5462, -3.9244) -> (34.5462, -5.6564)
  line L383 (31.5462, -3.9244) -> (32.5462, -2.1923)
  line L384 (32.5462, -2.1923) -> (34.5462, -2.1923)
  line L385 (34.5462, -2.1923) -> (35.5462, -3.9244)
  line L386 (37.2782, -8.3885) -> (36.2782, -6.6564)
  line L387 (40.2782, -6.6564) -> (39.2782, -8.3885)
  line L388 (37.2782, -4.9244) -> (39.2782, -4.9244)
  line L389 (39.2782, -4.9244) -> (40.2782, -6.6564)
  line L390 (39.2782, -8.3885) -> (37.2782, -8.3885)
  line L391 (36.2782, -6.6564) -> (37.2782, -4.9244)
  line L392 (42.0103, -5.6564) -> (41.0103, -3.9244)
  line L393 (44.0103, -5.6564) -> (42.0103, -5.6564)
  line L394 (45.0103, -3.9244) -> (44.0103, -5.6564)
  line L395 (41.0103, -3.9244) -> (42.0103, -2.1923)
  line L396 (42.0103, -2.1923) -> (44.0103, -2.1923)
  line L397 (44.0103, -2.1923) -> (45.0103, -3.9244)
  line L398 (46.7423, -8.3885) -> (45.7423, -6.6564)
  line L399 (49.7423, -6.6564) -> (48.7423, -8.3885)
  line L400 (46.7423, -4.9244) -> (48.7423, -4.9244)
  line L401 (48.7423, -4.9244) -> (49.7423, -6.6564)
  line L402 (48.7423, -8.3885) -> (46.7423, -8.3885)
  line L403 (45.7423, -6.6564) -> (46.7423, -4.9244)
  line L404 (51.4744, -5.6564) -> (50.4744, -3.9244)
  line L405 (53.4744, -5.6564) -> (51.4744, -5.6564)
  line L406 (54.4744, -3.9244) -> (53.4744, -5.6564)
  line L407 (50.4744, -3.9244) -> (51.4744, -2.1923)
  line L408 (51.4744, -2.1923) -> (53.4744, -2.1923)
  line L409 (53.4744, -2.1923) -> (54.4744, -3.9244)
  line L410 (56.2064, -8.3885) -> (55.2064, -6.6564)
  line L411 (59.2064, -6.6564) -> (58.2064, -8.3885)
  line L412 (56.2064, -4.9244) -> (58.2064, -4.9244)
  line L413 (58.2064, -4.9244) -> (59.2064, -6.6564)
  line L414 (58.2064, -8.3885) -> (56.2064, -8.3885)
  line L415 (55.2064, -6.6564) -> (56.2064, -4.9244)
  line L416 (60.9385, -5.6564) -> (59.9385, -3.9244)
  line L417 (62.9385, -5.6564) -> (60.9385, -5.6564)
  line L418 (63.9385, -3.9244) -> (62.9385, -5.6564)
  line L419 (59.9385, -3.9244) -> (60.9385, -2.1923)
  line L420 (60.9385, -2.1923) -> (62.9385, -2.1923)
  line L421 (62.9385, -2.1923) -> (63.9385, -3.9244)
  line L422 (65.6705, -8.3885) -> (64.6705, -6.6564)
  line L423 (68.6705, -6.6564) -> (67.6705, -8.3885)
  line L424 (65.6705, -4.9244) -> (67.6705, -4.9244)
  line L425 (67.6705, -4.9244) -> (68.6705, -6.6564)
  line L426 (67.6705, -8.3885) -> (65.6705, -8.3885)
  line L427 (64.6705, -6.6564) -> (65.6705, -4.9244)
  line L428 (70.4026, -5.6564) -> (69.4026, -3.9244)
  line L429 (72.4026, -5.6564) -> (70.4026, -5.6564)
  line L430 (73.4026, -3.9244) -> (72.4026, -5.6564)
  line L431 (69.4026, -3.9244) -> (70.4026, -2.1923)
  line L432 (70.4026, -2.1923) -> (72.4026, -2.1923)
  line L433 (72.4026, -2.1923) -> (73.4026, -3.9244)
  line L434 (75.1346, -8.3885) -> (74.1346, -6.6564)
  line L435 (78.1346, -6.6564) -> (77.1346, -8.3885)
  line L436 (75.1346, -4.9244) -> (77.1346, -4.9244)
  line L437 (77.1346, -4.9244) -> (78.1346, -6.6564)
  line L438 (77.1346, -8.3885) -> (75.1346, -8.3885)
  line L439 (74.1346, -6.6564) -> (75.1346, -4.9244)
  line L440 (79.8667, -5.6564) -> (78.8667, -3.9244)
  line L441 (81.8667, -5.6564) -> (79.8667, -5.6564)
  line L442 (82.8667, -3.9244) -> (81.8667, -5.6564)
  line L443 (78.8667, -3.9244) -> (79.8667, -2.1923)
  line L444 (79.8667, -2.1923) -> (81.8667, -2.1923)
  line L445 (81.8667, -2.1923) -> (82.8667, -3.9244)
  line L446 (18.35, -13.8526) -> (17.35, -12.1205)
  line L447 (21.35, -12.1205) -> (20.35, -13.8526)
  line L448 (18.35, -10.3885) -> (20.35, -10.3885)
  line L449 (20.35, -10.3885) -> (21.35, -12.1205)
  line L450 (20.35, -13.8526) -> (18.35, -13.8526)
  line L451 (17.35, -12.1205) -> (18.35, -10.3885)
  line L452 (23.0821, -11.1205) -> (22.0821, -9.3885)
  line L453 (25.0821, -11.1205) -> (23.0821, -11.1205)
  line L454 (26.0821, -9.3885) -> (25.0821, -11.1205)
  line L455 (22.0821, -9.3885) -> (23.0821, -7.6564)
  line L456 (23.0821, -7.6564) -> (25.0821, -7.6564)
  line L457 (25.0821, -7.6564) -> (26.0821, -9.3885)
  line L458 (27.8141, -13.8526) -> (26.8141, -12.1205)
  line L459 (30.8141, -12.1205) -> (29.8141, -13.8526)
  line L460 (27.8141, -10.3885) -> (29.8141, -10.3885)
  line L461 (29.8141, -10.3885) -> (30.8141, -12.1205)
  line L462 (29.8141, -13.8526) -> (27.8141, -13.8526)
  line L463 (26.8141, -12.1205) -> (27.8141, -10.3885)
  line L464 (32.5462, -11.1205) -> (31.5462, -9.3885)
  line L465 (34.5462, -11.1205) -> (32.5462, -11.1205)
  line L466 (35.5462, -9.3885) -> (34.5462, -11.1205)
  line L467 (31.5462, -9.3885) -> (32.5462, -7.6564)
  line L468 (32.5462, -7.6564) -> (34.5462, -7.6564)
  line L469 (34.5462, -7.6564) -> (35.5462, -9.3885)
  line L470 (37.2782, -13.8526) -> (36.2782, -12.1205)
  line L471 (40.2782, -12.1205) -> (39.2782, -13.8526)
  line L472 (37.2782, -10.3885) -> (39.2782, -10.3885)
  line L473 (39.2782, -10.3885) -> (40.2782, -12.1205)
  line L474 (39.2782, -13.8526) -> (37.2782, -13.8526)
  line L475 (36.2782, -12.1205) -> (37.2782, -10.3885)
  line L476 (42.0103, -11.1205) -> (41.0103, -9.3885)
  line L477 (44.0103, -11.1205) -> (42.0103, -11.1205)
  line L478 (45.0103, -9.3885) -> (44.0103, -11.1205)
  line L479 (41.0103, -9.3885) -> (42.0103, -7.6564)
  line L480 (42.0103, -7.6564) -> (44.0103, -7.6564)
  line L481 (44.0103, -7.6564) -> (45.0103, -9.3885)
  line L482 (46.7423, -13.8526) -> (45.7423, -12.1205)
  line L483 (49.7423, -12.1205) -> (48.7423, -13.8526)
  line L484 (46.7423, -10.3885) -> (48.7423, -10.3885)
  line L485 (48.7423, -10.3885) -> (49.7423, -12.1205)
  line L486 (48.7423, -13.8526) -> (46.7423, -13.8526)
  line L487 (45.7423, -12.1205) -> (46.7423, -10.3885)
  line L488 (51.4744, -11.1205) -> (50.4744, -9.3885)
  line L489 (53.4744, -11.1205) -> (51.4744, -11.1205)
  line L490 (54.4744, -9.3885) -> (53.4744, -11.1205)
  line L491 (50.4744, -9.3885) -> (51.4744, -7.6564)
  line L492 (51.4744, -7.6564) -> (53.4744, -7.6564)
  line L493 (53.4744, -7.6564) -> (54.4744, -9.3885)
  line L494 (56.2064, -13.8526) -> (55.2064, -12.1205)
  line L495 (59.2064, -12.1205) -> (58.2064, -13.8526)
  line L496 (56.2064, -10.3885) -> (58.2064, -10.3885)
  line L497 (58.2064, -10.3885) -> (59.2064, -12.1205)
  line L498 (58.2064, -13.8526) -> (56.2064, -13.8526)
  line L499 (55.2064, -12.1205) -> (56.2064, -10.3885)
  line L500 (60.9385, -11.1205) -> (59.9385, -9.3885)
  line L501 (62.9385, -11.1205) -> (60.9385, -11.1205)
  line L502 (63.9385, -9.3885) -> (62.9385, -11.1205)
  line L503 (59.9385, -9.3885) -> (60.9385, -7.6564)
  line L504 (60.9385, -7.6564) -> (62.9385, -7.6564)
  line L505 (62.9385, -7.6564) -> (63.9385, -9.3885)
  line L506 (65.6705, -13.8526) -> (64.6705, -12.1205)
  line L507 (68.6705, -12.1205) -> (67.6705, -13.8526)
  line L508 (65.6705, -10.3885) -> (67.6705, -10.3885)
  line L509 (67.6705, -10.3885) -> (68.6705, -12.1205)
  line L510 (67.6705, -13.8526) -> (65.6705, -13.8526)
  line L511 (64.6705, -12.1205) -> (65.6705, -10.3885)
  line L512 (70.4026, -11.1205) -> (69.4026, -9.3885)
  line L513 (72.4026, -11.1205) -> (70.4026, -11.1205)
  line L514 (73.4026, -9.3885) -> (72.4026, -11.1205)
  line L515 (69.4026, -9.3885) -> (70.4026, -7.6564)
  line L516 (70.4026, -7.6564) -> (72.4026, -7.6564)
  line L517 (72.4026, -7.6564) -> (73.4026, -9.3885)
  line L518 (75.1346, -13.8526) -> (74.1346, -12.1205)
  line L519 (78.1346, -12.1205) -> (77.1346, -13.8526)
  line L520 (75.1346, -10.3885) -> (77.1346, -10.3885)
  line L521 (77.1346, -10.3885) -> (78.1346, -12.1205)
  line L522 (77.1346, -13.8526) -> (75.1346, -13.8526)
  line L523 (74.1346, -12.1205) -> (75.1346, -10.3885)
  line L524 (79.8667, -11.1205) -> (78.8667, -9.3885)
  line L525 (81.8667, -11.1205) -> (79.8667, -11.1205)
  line L526 (82.8667, -9.3885) -> (81.8667, -11.1205)
  line L527 (78.8667, -9.3885) -> (79.8667, -7.6564)
  line L528 (79.8667, -7.6564) -> (81.8667, -7.6564)
  line L529 (81.8667, -7.6564) -> (82.8667, -9.3885)
  line L530 (18.35, -19.3167) -> (17.35, -17.5846)
  line L531 (21.35, -17.5846) -> (20.35, -19.3167)
  line L532 (18.35, -15.8526) -> (20.35, -15.8526)
  line L533 (20.35, -15.8526) -> (21.35, -17.5846)
  line L534 (20.35, -19.3167) -> (18.35, -19.3167)
  line L535 (17.35, -17.5846) -> (18.35, -15.8526)
  line L536 (23.0821, -16.5846) -> (22.0821, -14.8526)
  line L537 (25.0821, -16.5846) -> (23.0821, -16.5846)
  line L538 (26.0821, -14.8526) -> (25.0821, -16.5846)
  line L539 (22.0821, -14.8526) -> (23.0821, -13.1205)
  line L540 (23.0821, -13.1205) -> (25.0821, -13.1205)
  line L541 (25.0821, -13.1205) -> (26.0821, -14.8526)
  line L542 (27.8141, -19.3167) -> (26.8141, -17.5846)
  line L543 (30.8141, -17.5846) -> (29.8141, -19.3167)
  line L544 (27.8141, -15.8526) -> (29.8141, -15.8526)
  line L545 (29.8141, -15.8526) -> (30.8141, -17.5846)
  line L546 (29.8141, -19.3167) -> (27.8141, -19.3167)
  line L547 (26.8141, -17.5846) -> (27.8141, -15.8526)
  line L548 (32.5462, -16.5846) -> (31.5462, -14.8526)
  line L549 (34.5462, -16.5846) -> (32.5462, -16.5846)
  line L550 (35.5462, -14.8526) -> (34.5462, -16.5846)
  line L551 (31.5462, -14.8526) -> (32.5462, -13.1205)
  line L552 (32.5462, -13.1205) -> (34.5462, -13.1205)
  line L553 (34.5462, -13.1205) -> (35.5462, -14.8526)
  line L554 (37.2782, -19.3167) -> (36.2782, -17.5846)
  line L555 (40.2782, -17.5846) -> (39.2782, -19.3167)
  line L556 (37.2782, -15.8526) -> (39.2782, -15.8526)
  line L557 (39.2782, -15.8526) -> (40.2782, -17.5846)
  line L558 (39.2782, -19.3167) -> (37.2782, -19.3167)
  line L559 (36.2782, -17.5846) -> (37.2782, -15.8526)
  line L560 (42.0103, -16.5846) -> (41.0103, -14.8526)
  line L561 (44.0103, -16.5846) -> (42.0103, -16.5846)
  line L562 (45.0103, -14.8526) -> (44.0103, -16.5846)
  line L563 (41.0103, -14.8526) -> (42.0103, -13.1205)
  line L564 (42.0103, -13.1205) -> (44.0103, -13.1205)
  line L565 (44.0103, -13.1205) -> (45.0103, -14.8526)
  line L566 (46.7423, -19.3167) -> (45.7423, -17.5846)
  line L567 (49.7423, -17.5846) -> (48.7423, -19.3167)
  line L568 (46.7423, -15.8526) -> (48.7423, -15.8526)
  line L569 (48.7423, -15.8526) -> (49.7423, -17.5846)
  line L570 (48.7423, -19.3167) -> (46.7423, -19.3167)
  line L571 (45.7423, -17.5846) -> (46.7423, -15.8526)
  line L572 (51.4744, -16.5846) -> (50.4744, -14.8526)
  line L573 (53.4744, -16.5846) -> (51.4744, -16.5846)
  line L574 (54.4744, -14.8526) -> (53.4744, -16.5846)
  line L575 (50.4744, -14.8526) -> (51.4744, -13.1205)
  line L576 (51.4744, -13.1205) -> (53.4744, -13.1205)
  line L577 (53.4744, -13.1205) -> (54.4744, -14.8526)
  line L578 (56.2064, -19.3167) -> (55.2064, -17.5846)
  line L579 (59.2064, -17.5846) -> (58.2064, -19.3167)
  line L580 (56.2064, -15.8526) -> (58.2064, -15.8526)
  line L581 (58.2064, -15.8526) -> (59.2064, -17.5846)
  line L582 (58.2064, -19.3167) -> (56.2064, -19.3167)
  line L583 (55.2064, -17.5846) -> (56.2064, -15.8526)
  line L584 (60.9385, -16.5846) -> (59.9385, -14.8526)
  line L585 (62.9385, -16.5846) -> (60.9385, -16.5846)
  line L586 (63.9385, -14.8526) -> (62.9385, -16.5846)
  line L587 (59.9385, -14.8526) -> (60.9385, -13.1205)
  line L588 (60.9385, -13.1205) -> (62.9385, -13.1205)
  line L589 (62.9385, -13.1205) -> (63.9385, -14.8526)
  line L590 (65.6705, -19.3167) -> (64.6705, -17.5846)
  line L591 (68.6705, -17.5846) -> (67.6705, -19.3167)
  line L592 (65.6705, -15.8526) -> (67.6705, -15.8526)
  line L593 (67.6705, -15.8526) -> (68.6705, -17.5846)
  line L594 (67.6705, -19.3167) -> (65.6705, -19.3167)
  line L595 (64.6705, -17.5846) -> (65.6705, -15.8526)
  line L596 (70.4026, -16.5846) -> (69.4026, -14.8526)
  line L597 (72.4026, -16.5846) -> (70.4026, -16.5846)
  line L598 (73.4026, -14.8526) -> (72.4026, -16.5846)
  line L599 (69.4026, -14.8526) -> (70.4026, -13.1205)
  line L600 (70.4026, -13.1205) -> (72.4026, -13.1205)
  line L601 (72.4026, -13.1205) -> (73.4026, -14.8526)
  line L602 (75.1346, -19.3167) -> (74.1346, -17.5846)
  line L603 (78.1346, -17.5846) -> (77.1346, -19.3167)
  line L604 (75.1346, -15.8526) -> (77.1346, -15.8526)
  line L605 (77.1346, -15.8526) -> (78.1346, -17.5846)
  line L606 (77.1346, -19.3167) -> (75.1346, -19.3167)
  line L607 (74.1346, -17.5846) -> (75.1346, -15.8526)
  line L608 (79.8667, -16.5846) -> (78.8667, -14.8526)
  line L609 (81.8667, -16.5846) -> (79.8667, -16.5846)
  line L610 (82.8667, -14.8526) -> (81.8667, -16.5846)
  line L611 (78.8667, -14.8526) -> (79.8667, -13.1205)
  line L612 (79.8667, -13.1205) -> (81.8667, -13.1205)
  line L613 (81.8667, -13.1205) -> (82.8667, -14.8526)
  line L614 (18.35, -24.7808) -> (17.35, -23.0487)
  line L615 (21.35, -23.0487) -> (20.35, -24.7808)
  line L616 (18.35, -21.3167) -> (20.35, -21.3167)
  line L617 (20.35, -21.3167) -> (21.35, -23.0487)
  line L618 (20.35, -24.7808) -> (18.35, -24.7808)
  line L619 (17.35, -23.0487) -> (18.35, -21.3167)
  line L620 (23.0821, -22.0487) -> (22.0821, -20.3167)
  line L621 (25.0821, -22.0487) -> (23.0821, -22.0487)
  line L622 (26.0821, -20.3167) -> (25.0821, -22.0487)
  line L623 (22.0821, -20.3167) -> (23.0821, -18.5846)
  line L624 (23.0821, -18.5846) -> (25.0821, -18.5846)
  line L625 (25.0821, -18.5846) -> (26.0821, -20.3167)
  line L626 (27.8141, -24.7808) -> (26.8141, -23.0487)
  line L627 (30.8141, -23.0487) -> (29.8141, -24.7808)
  line L628 (27.8141, -21.3167) -> (29.8141, -21.3167)
  line L629 (29.8141, -21.3167) -> (30.8141, -23.0487)
  line L630 (29.8141, -24.7808) -> (27.8141, -24.7808)
  line L631 (26.8141, -23.0487) -> (27.8141, -21.3167)
  line L632 (32.5462, -22.0487) -> (31.5462, -20.3167)
  line L633 (34.5462, -22.0487) -> (32.5462, -22.0487)
  line L634 (35.5462, -20.3167) -> (34.5462, -22.0487)
  line L635 (31.5462, -20.3167) -> (32.5462, -18.5846)
  line L636 (32.5462, -18.5846) -> (34.5462, -18.5846)
  line L637 (34.5462, -18.5846) -> (35.5462, -20.3167)
  line L638 (37.2782, -24.7808) -> (36.2782, -23.0487)
  line L639 (40.2782, -23.0487) -> (39.2782, -24.7808)
  line L640 (37.2782, -21.3167) -> (39.2782, -21.3167)
  line L641 (39.2782, -21.3167) -> (40.2782, -23.0487)
  line L642 (39.2782, -24.7808) -> (37.2782, -24.7808)
  line L643 (36.2782, -23.0487) -> (37.2782, -21.3167)
  line L644 (42.0103, -22.0487) -> (41.0103, -20.3167)
  line L645 (44.0103, -22.0487) -> (42.0103, -22.0487)
  line L646 (45.0103, -20.3167) -> (44.0103, -22.0487)
  line L647 (41.0103, -20.3167) -> (42.0103, -18.5846)
  line L648 (42.0103, -18.5846) -> (44.0103, -18.5846)
  line L649 (44.0103, -18.5846) -> (45.0103, -20.3167)
  line L650 (46.7423, -24.7808) -> (45.7423, -23.0487)
  line L651 (49.7423, -23.0487) -> (48.7423, -24.7808)
  line L652 (46.7423, -21.3167) -> (48.7423, -21.3167)
  line L653 (48.7423, -21.3167) -> (49.7423, -23.0487)
  line L654 (48.7423, -24.7808) -> (46.7423, -24.7808)
  line L655 (45.7423, -23.0487) -> (46.7423, -21.3167)
  line L656 (51.4744, -22.0487) -> (50.4744, -20.3167)
  line L657 (53.4744, -22.0487) -> (51.4744, -22.0487)
  line L658 (54.4744, -20.3167) -> (53.4744, -22.0487)
  line L659 (50.4744, -20.3167) -> (51.4744, -18.5846)
  line L660 (51.4744, -18.5846) -> (53.4744, -18.5846)
  line L661 (53.4744, -18.5846) -> (54.4744, -20.3167)
  line L662 (56.2064, -24.7808) -> (55.2064, -23.0487)
  line L663 (59.2064, -23.0487) -> (58.2064, -24.7808)
  line L664 (56.2064, -21.3167) -> (58.2064, -21.3167)
  line L665 (58.2064, -21.3167) -> (59.2064, -23.0487)
  line L666 (58.2064, -24.7808) -> (56.2064, -24.7808)
  line L667 (55.2064, -23.0487) -> (56.2064, -21.3167)
  line L668 (60.9385, -22.0487) -> (59.9385, -20.3167)
  line L669 (62.9385, -22.0487) -> (60.9385, -22.0487)
  line L670 (63.9385, -20.3167) -> (62.9385, -22.0487)
  line L671 (59.9385, -20.3167) -> (60.9385, -18.5846)
  line L672 (60.9385, -18.5846) -> (62.9385, -18.5846)
  line L673 (62.9385, -18.5846) -> (63.9385, -20.3167)
  line L674 (65.6705, -24.7808) -> (64.6705, -23.0487)
  line L675 (68.6705, -23.0487) -> (67.6705, -24.7808)
  line L676 (65.6705, -21.3167) -> (67.6705, -21.3167)
  line L677 (67.6705, -21.3167) -> (68.6705, -23.0487)
  line L678 (67.6705, -24.7808) -> (65.6705, -24.7808)
  line L679 (64.6705, -23.0487) -> (65.6705, -21.3167)
  line L680 (70.4026, -22.0487) -> (69.4026, -20.3167)
  line L681 (72.4026, -22.0487) -> (70.4026, -22.0487)
  line L682 (73.4026, -20.3167) -> (72.4026, -22.0487)
  line L683 (69.4026, -20.3167) -> (70.4026, -18.5846)
  line L684 (70.4026, -18.5846) -> (72.4026, -18.5846)
  line L685 (72.4026, -18.5846) -> (73.4026, -20.3167)
  line L686 (75.1346, -24.7808) -> (74.1346, -23.0487)
  line L687 (78.1346, -23.0487) -> (77.1346, -24.7808)
  line L688 (75.1346, -21.3167) -> (77.1346, -21.3167)
  line L689 (77.1346, -21.3167) -> (78.1346, -23.0487)
  line L690 (77.1346, -24.7808) -> (75.1346, -24.7808)
  line L691 (74.1346, -23.0487) -> (75.1346, -21.3167)
  line L692 (79.8667, -22.0487) -> (78.8667, -20.3167)
  line L693 (81.8667, -22.0487) -> (79.8667, -22.0487)
  line L694 (82.8667, -20.3167) -> (81.8667, -22.0487)
  line L695 (78.8667, -20.3167) -> (79.8667, -18.5846)
  line L696 (79.8667, -18.5846) -> (81.8667, -18.5846)
  line L697 (81.8667, -18.5846) -> (82.8667, -20.3167)
  line L698 (18.35, -30.2449) -> (17.35, -28.5128)
  line L699 (21.35, -28.5128) -> (20.35, -30.2449)
  line L700 (18.35, -26.7808) -> (20.35, -26.7808)
  line L701 (20.35, -26.7808) -> (21.35, -28.5128)
  line L702 (20.35, -30.2449) -> (18.35, -30.2449)
  line L703 (17.35, -28.5128) -> (18.35, -26.7808)
  line L704 (23.0821, -27.5128) -> (22.0821, -25.7808)
  line L705 (25.0821, -27.5128) -> (23.0821, -27.5128)
  line L706 (26.0821, -25.7808) -> (25.0821, -27.5128)
  line L707 (22.0821, -25.7808) -> (23.0821, -24.0487)
  line L708 (23.0821, -24.0487) -> (25.0821, -24.0487)
  line L709 (25.0821, -24.0487) -> (26.0821, -25.7808)
  line L710 (27.8141, -30.2449) -> (26.8141, -28.5128)
  line L711 (30.8141, -28.5128) -> (29.8141, -30.2449)
  line L712 (27.8141, -26.7808) -> (29.8141, -26.7808)
  line L713 (29.8141, -26.7808) -> (30.8141, -28.5128)
  line L714 (29.8141, -30.2449) -> (27.8141, -30.2449)
  line L715 (26.8141, -28.5128) -> (27.8141, -26.7808)
  line L716 (32.5462, -27.5128) -> (31.5462, -25.7808)
  line L717 (34.5462, -27.5128) -> (32.5462, -27.5128)
  line L718 (35.5462, -25.7808) -> (34.5462, -27.5128)
  line L719 (31.5462, -25.7808) -> (32.5462, -24.0487)
  line L720 (32.5462, -24.0487) -> (34.5462, -24.0487)
  line L721 (34.5462, -24.0487) -> (35.5462, -25.7808)
  line L722 (37.2782, -30.2449) -> (36.2782, -28.5128)
  line L723 (40.2782, -28.5128) -> (39.2782, -30.2449)
  line L724 (37.2782, -26.7808) -> (39.2782, -26.7808)
  line L725 (39.2782, -26.7808) -> (40.2782, -28.5128)
  line L726 (39.2782, -30.2449) -> (37.2782, -30.2449)
  line L727 (36.2782, -28.5128) -> (37.2782, -26.7808)
  line L728 (42.0103, -27.5128) -> (41.0103, -25.7808)
  line L729 (44.0103, -27.5128) -> (42.0103, -27.5128)
  line L730 (45.0103, -25.7808) -> (44.0103, -27.5128)
  line L731 (41.0103, -25.7808) -> (42.0103, -24.0487)
  line L732 (42.0103, -24.0487) -> (44.0103, -24.0487)
  line L733 (44.0103, -24.0487) -> (45.0103, -25.7808)
  line L734 (46.7423, -30.2449) -> (45.7423, -28.5128)
  line L735 (49.7423, -28.5128) -> (48.7423, -30.2449)
  line L736 (46.7423, -26.7808) -> (48.7423, -26.7808)
  line L737 (48.7423, -26.7808) -> (49.7423, -28.5128)
  line L738 (48.7423, -30.2449) -> (46.7423, -30.2449)
  line L739 (45.7423, -28.5128) -> (46.7423, -26.7808)
  line L740 (51.4744, -27.5128) -> (50.4744, -25.7808)
  line L741 (53.4744, -27.5128) -> (51.4744, -27.5128)
  line L742 (54.4744, -25.7808) -> (53.4744, -27.5128)
  line L743 (50.4744, -25.7808) -> (51.4744, -24.0487)
  line L744 (51.4744, -24.0487) -> (53.4744, -24.0487)
  line L745 (53.4744, -24.0487) -> (54.4744, -25.7808)
  line L746 (56.2064, -30.2449) -> (55.2064, -28.5128)
  line L747 (59.2064, -28.5128) -> (58.2064, -30.2449)
  line L748 (56.2064, -26.7808) -> (58.2064, -26.7808)
  line L749 (58.2064, -26.7808) -> (59.2064, -28.5128)
  line L750 (58.2064, -30.2449) -> (56.2064, -30.2449)
  line L751 (55.2064, -28.5128) -> (56.2064, -26.7808)
  line L752 (60.9385, -27.5128) -> (59.9385, -25.7808)
  line L753 (62.9385, -27.5128) -> (60.9385, -27.5128)
  line L754 (63.9385, -25.7808) -> (62.9385, -27.5128)
  line L755 (59.9385, -25.7808) -> (60.9385, -24.0487)
  line L756 (60.9385, -24.0487) -> (62.9385, -24.0487)
  line L757 (62.9385, -24.0487) -> (63.9385, -25.7808)
  line L758 (65.6705, -30.2449) -> (64.6705, -28.5128)
  line L759 (68.6705, -28.5128) -> (67.6705, -30.2449)
  line L760 (65.6705, -26.7808) -> (67.6705, -26.7808)
  line L761 (67.6705, -26.7808) -> (68.6705, -28.5128)
  line L762 (67.6705, -30.2449) -> (65.6705, -30.2449)
  line L763 (64.6705, -28.5128) -> (65.6705, -26.7808)
  line L764 (70.4026, -27.5128) -> (69.4026, -25.7808)
  line L765 (72.4026, -27.5128) -> (70.4026, -27.5128)
  line L766 (73.4026, -25.7808) -> (72.4026, -27.5128)
  line L767 (69.4026, -25.7808) -> (70.4026, -24.0487)
  line L768 (70.4026, -24.0487) -> (72.4026, -24.0487)
  line L769 (72.4026, -24.0487) -> (73.4026, -25.7808)
  line L770 (75.1346, -30.2449) -> (74.1346, -28.5128)
  line L771 (78.1346, -28.5128) -> (77.1346, -30.2449)
  line L772 (75.1346, -26.7808) -> (77.1346, -26.7808)
  line L773 (77.1346, -26.7808) -> (78.1346, -28.5128)
  line L774 (77.1346, -30.2449) -> (75.1346, -30.2449)
  line L775 (74.1346, -28.5128) -> (75.1346, -26.7808)
  line L776 (79.8667, -27.5128) -> (78.8667, -25.7808)
  line L777 (81.8667, -27.5128) -> (79.8667, -27.5128)
  line L778 (82.8667, -25.7808) -> (81.8667, -27.5128)
  line L779 (78.8667, -25.7808) -> (79.8667, -24.0487)
  line L780 (79.8667, -24.0487) -> (81.8667, -24.0487)
  line L781 (81.8667, -24.0487) -> (82.8667, -25.7808)
  line L782 (18.35, -35.709) -> (17.35, -33.9769)
  line L783 (21.35, -33.9769) -> (20.35, -35.709)
  line L784 (18.35, -32.2449) -> (20.35, -32.2449)
  line L785 (20.35, -32.2449) -> (21.35, -33.9769)
  line L786 (20.35, -35.709) -> (18.35, -35.709)
  line L787 (17.35, -33.9769) -> (18.35, -32.2449)
  line L788 (23.0821, -32.9769) -> (22.0821, -31.2449)
  line L789 (25.0821, -32.9769) -> (23.0821, -32.9769)
  line L790 (26.0821, -31.2449) -> (25.0821, -32.9769)
  line L791 (22.0821, -31.2449) -> (23.0821, -29.5128)
  line L792 (23.0821, -29.5128) -> (25.0821, -29.5128)
  line L793 (25.0821, -29.5128) -> (26.0821, -31.2449)
  line L794 (27.8141, -35.709) -> (26.8141, -33.9769)
  line L795 (30.8141, -33.9769) -> (29.8141, -35.709)
  line L796 (27.8141, -32.2449) -> (29.8141, -32.2449)
  line L797 (29.8141, -32.2449) -> (30.8141, -33.9769)
  line L798 (29.8141, -35.709) -> (27.8141, -35.709)
  line L799 (26.8141, -33.9769) -> (27.8141, -32.2449)
  line L800 (32.5462, -32.9769) -> (31.5462, -31.2449)
  line L801 (34.5462, -32.9769) -> (32.5462, -32.9769)
  line L802 (35.5462, -31.2449) -> (34.5462, -32.9769)
  line L803 (31.5462, -31.2449) -> (32.5462, -29.5128)
  line L804 (32.5462, -29.5128) -> (34.5462, -29.5128)
  line L805 (34.5462, -29.5128) -> (35.5462, -31.2449)
  line L806 (37.2782, -35.709) -> (36.2782, -33.9769)
  line L807 (40.2782, -33.9769) -> (39.2782, -35.709)
  line L808 (37.2782, -32.2449) -> (39.2782, -32.2449)
  line L809 (39.2782, -32.2449) -> (40.2782, -33.9769)